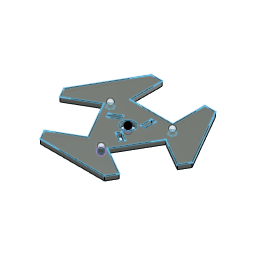
BottomTest v12 (Autodesk Fusion 360 archive; units mm, degrees)
design "BottomTest" references "StepperMount"
Autodesk Fusion 360 part; units mm, degrees
note: some values were not read from the file. Chosen so that the rebuilt part matches the saved one: which face or edge a step refers to; add or cut. Set by a fixed rule: which sketch regions a step uses.
imported_body "衍生的基础特征2" makes body 1
sketch "草图1" plane through (0, 0, 0) normal (0, 1, 0) x (1, 0, 0)
  line L0 (60, 0) -> (30, 51.9615)
  line L1 (-30, 51.9615) -> (-60, 0)
  line L2 (-30, -51.9615) -> (30, -51.9615)
  circle A0 centre (0, 0) radius 6
  line L3 (6, 6) -> (10, 6)
  line L4 (10, 6) -> (10, 16)
  line L5 (10, 16) -> (6, 16)
  line L6 (6, 16) -> (6, 6)
  circle A1 centre (-27.5, 11) radius 1.5
  line L7 (-18.8564, 0.6603) -> (-16.8564, -2.8038)
  line L8 (-16.8564, -2.8038) -> (-8.1962, 2.1962)
  line L9 (-8.1962, 2.1962) -> (-10.1962, 5.6603)
  circle A2 centre (4.2237, -29.3157) radius 1.5
  line L10 (-10.1962, 5.6603) -> (-18.8564, 0.6603)
  line L11 (8.8564, -16.6603) -> (10.8564, -13.1962)
  line L12 (10.8564, -13.1962) -> (2.1962, -8.1962)
  line L13 (2.1962, -8.1962) -> (0.1962, -11.6603)
  circle A3 centre (23.2763, 18.3157) radius 1.5
  line L14 (0.1962, -11.6603) -> (8.8564, -16.6603)
  line L15 (20, 22) -> (20, 51.9615)
  line L16 (-20, 22) -> (-20, 51.9615)
  line L17 (30, 51.9615) -> (20, 51.9615)
  line L18 (-20, 51.9615) -> (-30, 51.9615)
  line L19 (-20, 22) -> (20, 22)
  line L20 (-29.0526, 6.3205) -> (-55, -8.6603)
  line L21 (-9.0526, -28.3205) -> (-35, -43.3013)
  line L22 (-9.0526, -28.3205) -> (-29.0526, 6.3205)
  line L23 (9.0526, -28.3205) -> (35, -43.3013)
  line L24 (29.0526, 6.3205) -> (55, -8.6603)
  line L25 (29.0526, 6.3205) -> (9.0526, -28.3205)
  line L26 (30, -51.9615) -> (35, -43.3013)
  line L27 (55, -8.6603) -> (60, 0)
  line L28 (-60, 0) -> (-55, -8.6603)
  line L29 (-35, -43.3013) -> (-30, -51.9615)
  dimension "d23" = 3
  dimension "d25" = 360
  dimension "d27" = 360
  constraint coincident A0.centre origin
  constraint horizontal L3
  constraint vertical L4
  constraint horizontal L5
  constraint vertical L6
  constraint perpendicular L15 L17
  constraint coincident L16.end L17
  constraint perpendicular L16 L17
  constraint collinear L17 L18
  constraint perpendicular L15 L19
  constraint collinear L26 L27
  constraint collinear L28 L29
  measures "d23" diameter of A1
imported_body "衍生的基础特征1" makes body 2
move_body "移动1" bodies 2 to x (1, 0, 0) y (0, 1, 0) z (0, 0, 1) at (0, -0.1156, -5.9989)
copy_body "复制和粘贴实体1" bodies 2 makes body 3
move_body "移动2" bodies 3 to x (0, 0, -1) y (0, 1, 0) z (1, 0, 0) at (-0.0011, 0, 0.0011)
copy_body "复制和粘贴实体2" bodies 2 makes body 4
move_body "移动3" bodies 4 to x (0.866025, 0, 0.5) y (0, 1, 0) z (-0.5, 0, 0.866025) at (0.0006, 0, 0.0001)
move_body "移动4" bodies 2 to x (-0.866025, 0, 0.5) y (0, 1, 0) z (-0.5, 0, -0.866025) at (0.0006, 0, 0.0021)
move_body "移动5" bodies 3 to x (1, 0, 0) y (0, 1, 0) z (0, 0, 1) at (6, 0, 0)
move_body "移动6" bodies 4 to x (1, 0, 0) y (0, 1, 0) z (0, 0, 1) at (-3, 0, 5.1962)
move_body "移动7" bodies 2 to x (1, 0, 0) y (0, 1, 0) z (0, 0, 1) at (-3, 0, -5.1962)
move_body "移动8" bodies 3 to x (1, 0, 0) y (0, 1, 0) z (0, 0, 1) at (0, 0, -6)
move_body "移动9" bodies 4 to x (1, 0, 0) y (0, 1, 0) z (0, 0, 1) at (5.1962, 0, 3)
move_body "移动10" bodies 2 to x (1, 0, 0) y (0, 1, 0) z (0, 0, 1) at (-5.1962, 0, 3)
other "外部衍生2"
move_body "移动12" bodies 1 to x (1, 0, 0) y (0, 0, 1) z (0, -1, 0) at (0, 0, 0)
move_body "移动13" bodies 1 to x (-1, 0, 0) y (0, 1, 0) z (0, 0, -1) at (-26, 0, 20)
move_body "移动14" bodies 1 to x (1, 0, 0) y (0, 1, 0) z (0, 0, 1) at (19, 1, -26)
extrude "拉伸2" cut sketch "草图1" against normal blind 4 bodies 2 3 4
extrude "拉伸3" cut sketch "草图1" against normal blind 4 bodies 2 3 4 1
delete_body "移除实体1" bodies 2
extrude "拉伸4" add sketch "草图1" against normal blind 4 separate body makes body 5
sketch "草图2" plane through (0, -4, 0) normal (0, -1, 0) x (1, 0, 0)
  circle A0 centre (23.2763, -18.3157) radius 1.5
  line L0 (0.1962, 11.6603) -> (8.8564, 16.6603)
  line L1 (8.8564, 16.6603) -> (10.8564, 13.1962)
  line L2 (10.8564, 13.1962) -> (2.1962, 8.1962)
  line L3 (2.1962, 8.1962) -> (0.1962, 11.6603)
  circle A1 centre (-27.5, -11) radius 1.5
  line L4 (-10.1962, -5.6603) -> (-18.8564, -0.6603)
  line L5 (-18.8564, -0.6603) -> (-16.8564, 2.8038)
  line L6 (-16.8564, 2.8038) -> (-8.1962, -2.1962)
  line L7 (-8.1962, -2.1962) -> (-10.1962, -5.6603)
  circle A2 centre (4.2237, 29.3157) radius 1.5
  circle A3 centre (0, 0) radius 6
  line L8 (6, -16) -> (6, -6)
  line L9 (6, -6) -> (10, -6)
  line L10 (10, -6) -> (10, -16)
  line L11 (10, -16) -> (6, -16)
  line L12 (-35, 43.3013) -> (-9.0526, 28.3205)
  line L13 (-9.0526, 28.3205) -> (-29.0526, -6.3205)
  line L14 (-29.0526, -6.3205) -> (-55, 8.6603)
  line L15 (-55, 8.6603) -> (-60, 0)
  line L16 (-60, 0) -> (-30, -51.9615)
  line L17 (-30, -51.9615) -> (-20, -51.9615)
  line L18 (-20, -51.9615) -> (-20, -22)
  line L19 (-20, -22) -> (20, -22)
  line L20 (20, -22) -> (20, -51.9615)
  line L21 (20, -51.9615) -> (30, -51.9615)
  line L22 (30, -51.9615) -> (60, 0)
  line L23 (60, 0) -> (55, 8.6603)
  line L24 (55, 8.6603) -> (29.0526, -6.3205)
  line L25 (29.0526, -6.3205) -> (9.0526, 28.3205)
  line L26 (9.0526, 28.3205) -> (35, 43.3013)
  line L27 (35, 43.3013) -> (30, 51.9615)
  line L28 (30, 51.9615) -> (-30, 51.9615)
  line L29 (-30, 51.9615) -> (-35, 43.3013)
  line L30 (7.1737, 29.3157) -> (5.6987, 31.8705)
  line L31 (5.6987, 31.8705) -> (2.7487, 31.8705)
  line L32 (2.7487, 31.8705) -> (1.2737, 29.3157)
  line L33 (1.2737, 29.3157) -> (2.7487, 26.7609)
  line L34 (2.7487, 26.7609) -> (5.6987, 26.7609)
  line L35 (5.6987, 26.7609) -> (7.1737, 29.3157)
  line L36 (-28.975, -8.4452) -> (-30.45, -11)
  line L37 (-30.45, -11) -> (-28.975, -13.5548)
  line L38 (-28.975, -13.5548) -> (-26.025, -13.5548)
  line L39 (-26.025, -13.5548) -> (-24.55, -11)
  line L40 (-24.55, -11) -> (-26.025, -8.4452)
  line L41 (-26.025, -8.4452) -> (-28.975, -8.4452)
  line L42 (21.8013, -20.8705) -> (24.7513, -20.8705)
  line L43 (24.7513, -20.8705) -> (26.2263, -18.3157)
  line L44 (26.2263, -18.3157) -> (24.7513, -15.7609)
  line L45 (24.7513, -15.7609) -> (21.8013, -15.7609)
  line L46 (21.8013, -15.7609) -> (20.3263, -18.3157)
  line L47 (20.3263, -18.3157) -> (21.8013, -20.8705)
  point P0 (4.2237, 29.3157)
  point P1 (4.2237, 29.3157)
  dimension "d34" = 2.95
  dimension "d38" = 360
  constraint coincident P1 P0
  measures "d34" distance of L30.start P1
extrude "拉伸5" cut sketch "草图2" against normal blind 2.5 contours L30 L31 L32 L33 L34 L35 bodies 5
extrude "拉伸6" cut sketch "草图2" against normal blind 2.5 contours L36 L37 L38 L39 L40 L41 bodies 5
extrude "拉伸7" cut sketch "草图2" against normal blind 2.5 contours L42 L43 L44 L45 L46 L47 bodies 5
named bodies: "实体1", "实体1 (1)", "实体1 (1) (1)", "实体1 (1) (1) (1)"

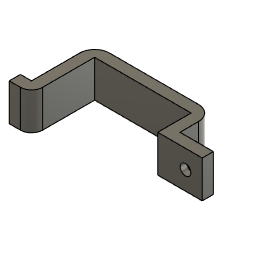
design "StepperMount"
Autodesk Fusion 360 part; units mm, degrees
sketch "草图1" plane through (0, 0, 0) normal (0, 1, 0) x (1, 0, 0)
  line L0 (12, 9) -> (38, 9)
  line L1 (38, 9) -> (38, 0)
  line L2 (38, 0) -> (50, 0)
  line L3 (50, 0) -> (50, 3)
  line L4 (50, 3) -> (41, 3)
  line L5 (41, 3) -> (41, 8)
  line L6 (37, 12) -> (13, 12)
  line L7 (9, -8) -> (6, -8)
  line L8 (6, -8) -> (6, -5)
  line L9 (6, -5) -> (9, -5)
  line L10 (9, 8) -> (9, -5)
  line L11 (12, 9) -> (12, -5)
  arc A0 (9, -8) -> (12, -5) centre (9, -5) ccw
  arc A1 (13, 12) -> (9, 8) centre (13, 8) ccw
  arc A2 (41, 8) -> (37, 12) centre (37, 8) ccw
  dimension "d21" = 3
  dimension "d22" = 4
  constraint perpendicular L0 L1
  constraint perpendicular L1 L2
  constraint perpendicular L2 L3
  constraint perpendicular L3 L4
  constraint perpendicular L4 L5
  constraint perpendicular L5 L6
  constraint perpendicular L7 L8
  constraint perpendicular L8 L9
  constraint perpendicular L9 L10
  constraint perpendicular L0 L11
  constraint tangent L7 A0
  constraint tangent L11 A0
  constraint tangent L6 A1
  constraint tangent L10 A1
  constraint tangent L5 A2
  constraint tangent L6 A2
  constraint equal A1 A2
  measures "d21" radius of A0
  measures "d22" radius of A1
extrude "拉伸1" add sketch "草图1" along normal blind 10
sketch "草图2" plane through (0, 0, -3) normal (0, 0, -1) x (-1, 0, 0)
  line L0 (-9, 0) -> (0, 0)
  line L1 (0, 0) -> (0, 10)
  line L2 (0, 10) -> (-9, 10)
  line L3 (-9, 10) -> (-9, 0)
  circle A0 centre (-4.5, 5) radius 1.5
  dimension "d3" = 3
  measures "d3" diameter of A0
hole "孔1" at (4.5, 5, -3) direction (0, 0, 1) diameter 3 depth 9 tip angle 180
hole "孔2" at (45.5, 5, -3) direction (0, 0, 1) diameter 2.9 depth 10 tip angle 180 countersink diameter 5.3 countersink angle 90
delete_face "删除面1" [no effect]
move_body "移动1" bodies 1 to x (1, 0, 0) y (0, 1, 0) z (0, 0, 1) at (-25, 0, 0)
hole "孔3" at (-20.5, 5, -3) direction (0, 0, 1) diameter 2.9 depth 10 tip angle 180 countersink diameter 5.3 countersink angle 90
